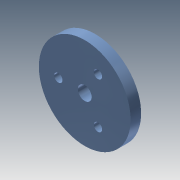
# Autodesk Inventor part: kolecko_rameno(2)
Saved by Autodesk Inventor 2013 (Build 170138000, 138)
## iProperties
Created: 2013-05-25
Part Number: kolecko_rameno(2)
Material: Generic
Document SubType Name: Modeling
Designer: idle-rug
Density: 1 g/cm^3
Author: idle-rug
Autodesk Inventor part; units mm, degrees
ref_plane "YZ Plane" through (0, 0, 0) normal (1, 0, 0) x (0, 1, 0)
ref_plane "XZ Plane" through (0, 0, 0) normal (0, 1, 0) x (-1, 0, 0)
ref_plane "XY Plane" through (0, 0, 0) normal (0, 0, 1) x (1, 0, 0)
sketch "Sketch1" plane through (0, 0, 0) normal (0, 1, 0) x (-1, 0, 0)
  circle A0 centre (0, 0) radius 16.575
  circle A1 centre (0, 0) radius 2.5
  dimension "d0" = 33.15
  dimension "d1" = 5
  constraints: 2 centre point, 2 coincident
  measures "d0" diameter of A0
  measures "d1" diameter of A1
extrude "Extrusion1" add sketch "Sketch1" along normal blind 3.8
sketch "Sketch2" plane through (0, 3.8, 0) normal (0, 1, 0) x (1, 0, 0)
  circle A0 centre (0, 0) radius 2.5 projected
  circle A1 centre (0, 0) radius 16.575 projected
  line L0 (-2.5, 0) -> (-16.575, 0)
  circle A2 centre (-9.5375, 0) radius 1.5
  line L1 (0, 0) -> (16.575, 0) construction
  line L2 (0, 0) -> (16.575, 0) construction
  circle A3 centre (4.7688, 8.2597) radius 1.5
  circle A4 centre (4.7688, -8.2597) radius 1.5
  dimension "d4" = 3
  dimension "d7" = 3
  dimension "d8" = 3
  constraints: 6 end point, 3 centre point, 3 horizontal, 2 horizontal alignment, 1 midpoint, 2 other
  measures "d4" diameter of A2
  measures "d7" diameter of A3
  measures "d8" diameter of A4
extrude "Extrusion2" cut sketch "Sketch2" against normal blind 3.8 contours A2 L0 | L0 A2 | A3 | A4
body "Solid1"
